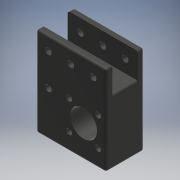
# Autodesk Inventor part: bed_pulley_holder
Saved by Autodesk Inventor 2018 (Build 220112000, 112)
## iProperties
Created: 2018-05-24
Part Number: bed_pulley_holder
Material: Plastic, Opaque Black
Document SubType Name: Modeling
Designer: Z. Deniz
Density: 0.952 g/cm^3
Appearance: Smooth - Black
Author: Z. Deniz
Autodesk Inventor part; units mm, degrees
ref_plane "YZ Plane" through (0, 0, 0) normal (1, 0, 0) x (0, 1, 0)
ref_plane "XZ Plane" through (0, 0, 0) normal (0, 1, 0) x (-1, 0, 0)
ref_plane "XY Plane" through (0, 0, 0) normal (0, 0, 1) x (1, 0, 0)
sketch "Sketch1" plane through (0, 0, 0) normal (0, 1, 0) x (-1, 0, 0)
  line L0 (-2, 0) -> (-30, 0)
  line L1 (-32, -2) -> (-32, -30)
  line L2 (-30, -32) -> (-2, -32)
  line L3 (0, -30) -> (0, -2)
  circle A0 centre (-16, -16) radius 10.5
  line L4 (1.5, -41) -> (-33.5, -41)
  line L5 (-33.5, -41) -> (-33.5, 9)
  line L6 (-33.5, 9) -> (1.5, 9)
  line L7 (1.5, 9) -> (1.5, -41)
  line L8 (1.5, -41) -> (-33.5, 9) construction
  line L9 (-33.5, -41) -> (1.5, 9) construction
  circle A1 centre (-16, -16) radius 16 construction
  line L10 (-2, -32) -> (0, -30)
  line L11 (0, -2) -> (-2, 0)
  line L12 (-30, 0) -> (-32, -2)
  line L13 (-30, -32) -> (-32, -30)
  line L14 (-16, -16) -> (0, 0) construction
  line L15 (-16, -16) -> (-32, 0) construction
  line L16 (-16, -16) -> (-32, -32) construction
  circle A2 centre (-27.3137, -27.3137) radius 2.25
  line L17 (-16, -16) -> (0, -32) construction
  circle A3 centre (-4.6863, -27.3137) radius 2.25
  circle A4 centre (-4.6863, -4.6863) radius 2.25
  circle A5 centre (-27.3137, -4.6863) radius 2.25
  line L18 (1.5, -41) -> (21.5, -41)
  line L19 (21.5, -41) -> (21.5, -21.5)
  line L20 (21.5, -21.5) -> (1.5, -21.5)
  line L21 (1.5, -21.5) -> (1.5, -41)
  dimension "d0" = 32
  dimension "d1" = 32
  dimension "d2" = 21
  dimension "d3" = 16
  dimension "d4" = 16
  dimension "d5" = 35
  dimension "d6" = 50
  dimension "d10" = 32
  dimension "d15" = 2
  dimension "d16" = 2
  dimension "d17" = 2
  dimension "d18" = 2
  dimension "d19" = 2
  dimension "d20" = 2
  dimension "d21" = 2
  dimension "d22" = 2
  dimension "d56" = 4.5
  dimension "d57" = 4.5
  dimension "d58" = 4.5
  dimension "d59" = 4.5
  dimension "d63" = 20
  dimension "d64" = 19.5
  constraints: 44 end point, 12 point on line, 6 centre point, 6 parallel, 4 perpendicular, 4 point on circle, 3 horizontal, 2 midpoint, 1 coincident
  measures "d0" distance of L17.end L16.end
  measures "d1" distance of L16.end point (-32, 0)
  measures "d2" diameter of A0
  measures "d3" distance from line of L3 A0.centre
  measures "d4" distance from line of L0 A0.centre
  measures "d5" distance of L5.end L6.end
  measures "d6" distance of L4.end L5.end
  measures "d10" diameter of A1
  measures "d15" distance of L2.end L17.end
  measures "d16" distance of L3.start L17.end
  measures "d17" distance of L3.end L14.end
  measures "d18" distance of L0.start L14.end
  measures "d19" distance of L0.end point (-32, 0)
  measures "d20" distance of L1.start point (-32, 0)
  measures "d21" distance of L2.start L16.end
  measures "d22" distance of L1.end L16.end
  measures "d56" diameter of A2
  measures "d57" diameter of A3
  measures "d58" diameter of A4
  measures "d59" diameter of A5
  measures "d63" distance of L20.end L19.end
  measures "d64" distance of L19.end L18.end
extrude "Extrusion1" add sketch "Sketch1" along normal blind 30 contours L11 L3 L10 L2 L13 L1 L12 L0 | L4 L5 L6 L7
sketch "Sketch3" plane through (-1.5, 0, 9) normal (0, 0, 1) x (1, 0, 0)
  line L0 (35, 0) -> (35, 30) projected
  line L1 (0, 0) -> (35, 0)
  line L2 (35, 0) -> (35, 5)
  line L3 (35, 5) -> (0, 5)
  line L4 (0, 5) -> (0, 0)
  point P0 (1.5, 0)
  dimension "d27" = 5
  constraints: 8 end point, 2 horizontal, 2 parallel, 1 perpendicular, 1 point on line, 1 vertical
  measures "d27" distance of L2.end L1.end
extrude "Extrusion2" add sketch "Sketch3" along normal blind 20
sketch "Sketch4" plane through (-1.5, 0, -41) normal (-1, 0, 0) x (0, 0, 1)
  line L0 (0, 0) -> (0, 30) projected
  line L1 (50, 5) -> (70, 5) projected
  line L2 (0, 0) -> (70, 0)
  line L3 (70, 0) -> (70, 5)
  line L4 (70, 5) -> (0, 5)
  line L5 (0, 5) -> (0, 0)
  point P0 (41, 0)
  constraints: 8 end point, 2 parallel, 1 horizontal, 1 perpendicular
extrude "Extrusion3" add sketch "Sketch4" along normal blind 20
sketch "Sketch5" plane through (-1.5, 30, 9) normal (0, 0, 1) x (1, 0, 0)
  line L0 (35, 0) -> (0, 0) projected
  line L1 (0, -25) -> (0, 0) projected
  line L2 (35, 0) -> (0, 0)
  line L3 (0, 0) -> (0, -5)
  line L4 (0, -5) -> (35, -5)
  line L5 (35, -5) -> (35, 0)
  point P0 (1.5, -30)
  dimension "d33" = 5
  constraints: 8 end point, 2 parallel, 1 horizontal, 1 perpendicular, 1 point on line
  measures "d33" distance of L3.end L2.end
extrude "Extrusion4" add sketch "Sketch5" along normal blind 20
sketch "Sketch6" plane through (-1.5, 5, -41) normal (-1, 0, 0) x (0, 0, 1)
  line L0 (50, 20) -> (70, 20) projected
  line L1 (0, 0) -> (0, 25) projected
  line L2 (70, 20) -> (0, 20)
  line L3 (0, 20) -> (0, 25)
  line L4 (0, 25) -> (70, 25)
  line L5 (70, 25) -> (70, 20)
  point P0 (41, -5)
  constraints: 8 end point, 2 parallel, 1 horizontal, 1 perpendicular
extrude "Extrusion5" add sketch "Sketch6" along normal blind 20
sketch "Sketch7" plane through (0, 0, 0) normal (0, -1, 0) x (1, 0, 0)
  line L0 (-21.5, -41) -> (-21.5, 29) projected
  line L1 (-21.5, -41) -> (33.5, -41) projected
  circle A0 centre (-11.5, 19) radius 2.5
  line L2 (33.5, 29) -> (-21.5, 29) projected
  circle A1 centre (6, 19) radius 2.5
  circle A2 centre (23.5, 19) radius 2.5
  line L3 (33.5, -41) -> (33.5, 29) projected
  circle A3 centre (-11.5, -6) radius 2.5
  line L4 (-21.5, -41) -> (-1.5, -41)
  line L5 (-1.5, -41) -> (-1.5, -23)
  line L6 (-1.5, -23) -> (-21.5, -23)
  line L7 (-21.5, -23) -> (-21.5, -41)
  point P0 (0, 0)
  dimension "d41" = 5
  dimension "d42" = 10
  dimension "d43" = 10
  dimension "d44" = 5
  dimension "d45" = 5
  dimension "d46" = 10
  dimension "d47" = 10
  dimension "d48" = 5
  dimension "d49" = 10
  dimension "d51" = 17.5
  dimension "d52" = 10
  dimension "d60" = 25
  dimension "d61" = 20
  dimension "d62" = 18
  constraints: 8 end point, 4 centre point, 2 parallel, 1 horizontal, 1 perpendicular
  measures "d41" diameter of A0
  measures "d42" distance from line of L2 A0.centre
  measures "d43" distance from line of L0 A0.centre
  measures "d44" diameter of A1
  measures "d45" diameter of A2
  measures "d46" distance from line of L3 A2.centre
  measures "d47" distance from line of L2 A2.centre
  measures "d48" diameter of A3
  measures "d49" distance from line of L0 A3.centre
  measures "d51" distance of A2.centre A1.centre
  measures "d52" distance from line of A1.centre L2
  measures "d60" distance of A0.centre A3.centre
  measures "d61" distance of L6.end L5.end
  measures "d62" distance of L5.end L4.end
extrude "Extrusion6" cut sketch "Sketch7" against normal blind 30 contours A0 | A1 | A2 | A3
fillet "Fillet1" radius 2 17 edges at (33.5, 15, -41) (-21.5, 2.5, -41) (-21.5, 27.5, -41) (33.5, 15, 9) (33.5, 2.5, 29) (33.5, 27.5, 29) (-21.5, 27.5, 29) (-21.5, 2.5, 29) (-1.5, 15, 9) (33.5, 0, -6) (6, 0, 29) (-21.5, 0, -6) (6, 0, -41) (33.5, 30, -6) (6, 30, -41) (-21.5, 30, -6) (6, 30, 29)
extrude "Extrusion7" add sketch "Sketch1" along normal blind 25 contours L7 L20 L19 L18
fillet "Fillet2" radius 2 4 edges at (-21.5, 12.5, -41) (-21.5, 0, -31.25) (-11.5, 0, -41) (-21.5, 15, -21.5)
equation "\"d16\" = d15"
equation "\"d17\" = d15"
equation "\"d18\" = d17"
equation "\"d19\" = d15"
equation "\"d20\" = d19"
equation "\"d21\" = d15"
equation "\"d22\" = d21"
body "Solid1"
